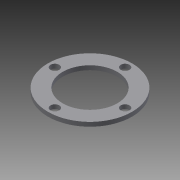
# Autodesk Inventor part: Hub 2
Saved by Autodesk Inventor 2013 (Build 170138000, 138)
## iProperties
Created: 2013-01-18
Part Number: Hub 2
Material: Generic
Document SubType Name: Sheet Metal
Designer: actoennies
Density: 1 g/cm^3
Sheet Metal Rule: Default
Mass: 5.37173 g
Surface Area: 46.9234 cm^2
Volume: 5.37173 cm^3
Author: actoennies
Autodesk Inventor part; units mm, degrees
ref_plane "YZ Plane" through (0, 0, 0) normal (1, 0, 0) x (0, 1, 0)
ref_plane "XZ Plane" through (0, 0, 0) normal (0, 1, 0) x (-1, 0, 0)
ref_plane "XY Plane" through (0, 0, 0) normal (0, 0, 1) x (1, 0, 0)
sketch "Sketch1" plane through (0, 0, 0) normal (0, 1, 0) x (-1, 0, 0)
  circle A0 centre (0, 0) radius 26.543 construction
  circle A1 centre (0, 26.543) radius 3.302
  circle A2 centre (26.543, 0) radius 3.302
  circle A3 centre (-26.543, 0) radius 3.302
  circle A4 centre (0, -26.543) radius 3.302
  circle A5 centre (0, 0) radius 20.6375
  circle A6 centre (0, 0) radius 31.75
  dimension "d0" = 53.086
  dimension "d1" = 6.604
  dimension "d2" = 6.604
  dimension "d3" = 6.604
  dimension "d4" = 6.604
  dimension "d5" = 41.275
  dimension "d6" = 63.5
  measures "d0" diameter of A0
  measures "d1" diameter of A1
  measures "d2" diameter of A2
  measures "d3" diameter of A3
  measures "d4" diameter of A4
  measures "d5" diameter of A5
  measures "d6" diameter of A6
extrude "Plate1" add sketch "Sketch1" along normal blind 3.175
equation "\"BendRadius\" = Thickness"
equation "\"BendReliefWidth\" = Thickness"
equation "\"BendReliefDepth\" = 0.5 * Thickness"
equation "\"CornerReliefSize\" = 4 * Thickness"
equation "\"MinimumRemnant\" = 2 * Thickness"
equation "\"TransitionRadius\" = BendRadius"
equation "\"JacobiRadiusSize\" = BendRadius"
equation "\"GapSize\" = Thickness"
equation "\"d7\" = BendRadius"
equation "\"Thickness\" = 3.175"
body "Solid1"
